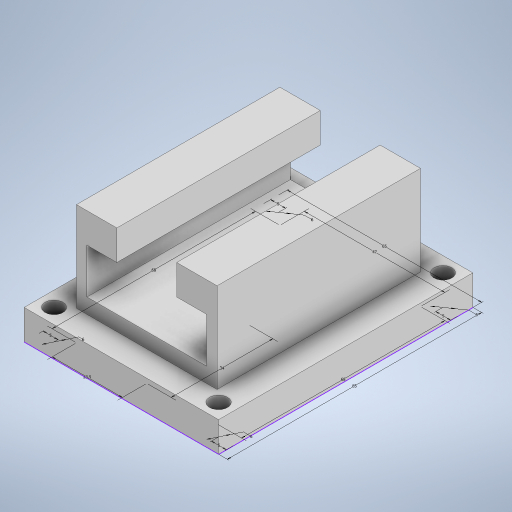
# Autodesk Inventor part: Base
Saved by Autodesk Inventor 2023 (Build 270158000, 158)
## iProperties
Created: 2022-06-21
Part Number: Base
Material: Generic
Document SubType Name: Modeling
Designer: nikol
Density: 1 g/cm^3
Appearance: Default
Author: nikol
Autodesk Inventor part; units mm, degrees
ref_plane "YZ Plane" through (0, 0, 0) normal (1, 0, 0) x (0, 1, 0)
ref_plane "XZ Plane" through (0, 0, 0) normal (0, 1, 0) x (-1, 0, 0)
ref_plane "XY Plane" through (0, 0, 0) normal (0, 0, 1) x (1, 0, 0)
sketch "Sketch1" plane through (0, 0, 0) normal (0, 1, 0) x (-1, 0, 0)
  point P0 (0, 0)
sketch "Sketch2" plane through (0, 0, 0) normal (0, 1, 0) x (-1, 0, 0)
  line L0 (10.9292, 17.7027) -> (-54.0708, 17.7027)
  line L1 (-54.0708, 17.7027) -> (-54.0708, -67.2973)
  line L2 (-54.0708, -67.2973) -> (10.9292, -67.2973)
  line L3 (10.9292, -67.2973) -> (10.9292, 17.7027)
  line L4 (10.9292, -24.7973) -> (-21.5708, -24.7973) construction
  line L5 (-21.5708, -24.7973) -> (-21.5708, 9.2027) construction
  line L6 (-21.5708, 9.2027) -> (1.9292, 9.2027)
  line L7 (1.9292, 9.2027) -> (1.9292, -58.7973)
  line L8 (1.9292, -58.7973) -> (-45.0708, -58.7973)
  line L9 (-45.0708, -58.7973) -> (-45.0708, 9.2027)
  line L10 (-45.0708, 9.2027) -> (-21.5708, 9.2027)
  line L11 (10.9292, 12.7027) -> (5.9292, 12.7027) construction
  circle A0 centre (5.9292, 12.7027) radius 3
  line L12 (10.9292, -62.2973) -> (5.9292, -62.2973) construction
  circle A1 centre (5.9292, -62.2973) radius 3
  line L13 (-54.0708, -62.2973) -> (-49.0708, -62.2973) construction
  circle A2 centre (-49.0708, -62.2973) radius 3
  line L14 (-54.0708, 12.7027) -> (-49.0708, 12.7027) construction
  circle A3 centre (-49.0708, 12.7027) radius 3
  point P0 (0, 0)
  dimension "d0" = 65
  dimension "d1" = 85
  dimension "d2" = 34
  dimension "d3" = 23.5
  dimension "d4" = 68
  dimension "d5" = 47
  dimension "d6" = 68
  dimension "d8" = 5
  dimension "d9" = 6
  dimension "d11" = 5
  dimension "d12" = 6
  dimension "d14" = 5
  dimension "d15" = 6
  dimension "d17" = 5
  dimension "d18" = 6
  constraints: 30 end point, 6 horizontal, 5 point on line, 4 centre point, 4 coincident, 4 perpendicular, 3 equal length, 1 midpoint, 1 vertical
  measures "d0" distance of L2.end L1.end
  measures "d1" distance of L1.end L0.end
  measures "d2" distance of L4.end L5.end
  measures "d3" distance of L5.end L6.end
  measures "d4" distance of L6.end L7.end
  measures "d5" distance of L7.end L8.end
  measures "d6" distance of L8.end L9.end
  measures "d8" distance of L11.start L11.end
  measures "d9" diameter of A0
  measures "d11" distance of L12.start L12.end
  measures "d12" diameter of A1
  measures "d14" distance of L13.start L13.end
  measures "d15" diameter of A2
  measures "d17" distance of L14.start L14.end
  measures "d18" diameter of A3
extrude "Extrusion1" add sketch "Sketch2" along normal blind 10 contours L3 L2 L1 L0 | L6 L7 L8 L9 L10
extrude "Extrusion2" cut sketch "Sketch2" along normal blind 20 contours L6 L7 L8 L9 L10
extrude "Extrusion3" add sketch "Sketch2" along normal blind 40 contours L6 L7 L8 L9 L10
sketch "Sketch3" plane through (45.0708, 10, -58.7973) normal (0, 0, -1) x (-1, 0, 0)
  line L0 (47, 30) -> (0, 30) projected
  line L1 (0, 30) -> (13.5, 30) construction
  line L2 (47, 30) -> (33.5, 30) construction
  line L3 (13.5, 30) -> (13.5, 20)
  line L4 (13.5, 20) -> (3.5, 20)
  line L5 (3.5, 20) -> (3.5, 5)
  line L6 (3.5, 5) -> (43.5, 5)
  line L7 (43.5, 5) -> (43.5, 20)
  line L8 (43.5, 20) -> (33.5, 20)
  line L9 (33.5, 20) -> (33.5, 30)
  line L10 (13.5, 30) -> (33.5, 30)
  point P0 (45.0708, -10)
  dimension "d25" = 13.5
  dimension "d26" = 13.5
  dimension "d27" = 10
  dimension "d28" = 10
  dimension "d29" = 15
  dimension "d30" = 40
  dimension "d31" = 15
  dimension "d32" = 10
  constraints: 20 end point, 4 perpendicular, 2 point on line, 2 vertical, 1 collinear
  measures "d25" distance of L0.end L1.end
  measures "d26" distance of L0.start L2.end
  measures "d27" distance of L1.end L3.end
  measures "d28" distance of L3.end L4.end
  measures "d29" distance of L4.end L5.end
  measures "d30" distance of L5.end L6.end
  measures "d31" distance of L6.end L7.end
  measures "d32" distance of L7.end L8.end
extrude "Extrusion4" cut sketch "Sketch3" against normal blind 68
body "Solid1"
